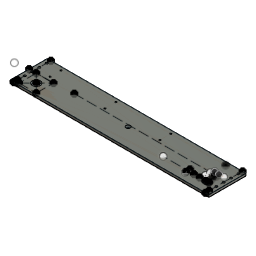
SideWall v52 (Autodesk Fusion 360 archive; units mm, degrees)
design "SideWall" references "tormach 770mx"
Autodesk Fusion 360 part; units mm, degrees
sketch "Sketch1" plane through (0, 0, 0) normal (0, 1, 0) x (1, 0, 0)
  line L0 (0, 0) -> (543, 0)
  line L1 (543, 0) -> (543, -101.6)
  line L2 (543, -101.6) -> (0, -101.6)
  line L3 (0, -101.6) -> (0, 0)
  dimension "d1" = 543
  dimension "d2" = 101.6
  constraint horizontal L0
  constraint vertical L1
  constraint horizontal L2
  constraint vertical L3
  constraint coincident L0.start L3.end
  measures "d1" distance of L0.start L0.end
  measures "d2" distance of L0.start L2.end
extrude "Extrude1" add sketch "Sketch1" along normal mid plane 6.35
sketch "Sketch2" plane through (0, 3.175, 0) normal (0, 1, 0) x (-1, 0, 0)
  line L0 (0, 101.6) -> (-543, 101.6)
  line L1 (-543, 101.6) -> (-543, 0)
  line L2 (-543, 0) -> (0, 0)
  line L3 (0, 0) -> (0, 101.6)
  line L4 (-534, 0) -> (-534, 101.6) construction
  line L5 (-10, 0) -> (-10, 101.6) construction
  line L6 (-506.5, 80.1) -> (-514.5, 80.1)
  arc A0 (-514.5, 80.1) -> (-514.5, 66.1) centre (-514.5, 73.1) ccw
  line L7 (-514.5, 66.1) -> (-506.5, 66.1)
  arc A1 (-506.5, 66.1) -> (-506.5, 80.1) centre (-506.5, 73.1) ccw
  line L8 (-506.5, 73.1) -> (-514.5, 73.1) construction
  line L9 (-506.5, 73.1) -> (-390, 73.1) construction
  line L10 (0, 49.6) -> (-66.57, 49.6) construction
  line L11 (-19.43, 96.67) -> (-66.57, 96.67) construction
  line L12 (-66.57, 96.67) -> (-66.57, 49.53) construction
  line L13 (-66.57, 49.53) -> (-19.43, 49.53) construction
  line L14 (-19.43, 49.53) -> (-19.43, 96.67) construction
  line L15 (-19.43, 96.67) -> (-66.57, 49.53) construction
  line L16 (-66.57, 96.67) -> (-19.43, 49.53) construction
  line L17 (-458, 67) -> (-458, 81) construction
  line L18 (-120, 46.09) -> (-504, 46.09) construction
  line L19 (-510, 47.46) -> (-510, 60.6) construction
  line L20 (-496.73, 39.09) -> (-522, 39.09) construction
  point P0 (-534, 91.6)
  point P1 (35, 55)
  point P2 (-10, 91.6)
  point P3 (-496.73, 9.09)
  point P4 (-496.73, 39.09)
  point P5 (-514.5, 73.1)
  point P6 (-506.5, 73.1)
  point P7 (-490, 73.1)
  point P8 (-474, 73.1)
  point P9 (-120, 46.09)
  point P10 (-504, 46.09)
  point P11 (-43, 73.1)
  point P12 (-19.43, 49.53)
  point P13 (-66.57, 49.53)
  point P14 (-66.57, 96.67)
  point P15 (-19.43, 96.67)
  point P16 (-458, 68.1)
  point P17 (-458, 78.1)
  point P18 (-508.73, 39.09)
  point P19 (-493, 60.6)
  point P20 (-493, 47.46)
  dimension "d6" = 10
  dimension "d14" = 10
  dimension "d15" = 10
  dimension "d27" = 30
  dimension "d40" = 8
  dimension "d42" = 28.5
  dimension "d43" = 14
  dimension "d45" = 16
  dimension "d46" = 490
  dimension "d47" = 506.5
  dimension "d48" = 534
  dimension "d49" = 496.73
  dimension "d50" = 92.51
  dimension "d68" = 52
  dimension "d69" = 120
  dimension "d70" = 504
  dimension "d77" = 47.14
  dimension "d78" = 47.14
  dimension "d79" = 43
  dimension "d80" = 28.5
  dimension "d102" = 10
  dimension "d103" = 16
  dimension "d104" = 5
  dimension "d112" = 55.51
  dimension "d114" = 510
  dimension "d115" = 13.14
  dimension "d122" = 41
  dimension "d123" = 12
  constraint coincident L2 L4.start
  constraint coincident L0 L4.end
  constraint perpendicular L0 L4
  constraint coincident L4 P0
  constraint coincident L2 L5.start
  constraint coincident L0 L5.end
  constraint perpendicular L0 L5
  constraint coincident L5 P2
  constraint horizontal P5 P6
  constraint tangent L6 A0
  constraint tangent A0 L7
  constraint parallel L6 L7
  constraint tangent L7 A1
  constraint tangent L6 A1
  constraint coincident P5 A0.centre
  constraint horizontal L8
  constraint coincident P6 A1.centre
  constraint parallel L8 L9
  constraint coincident L9 P7
  constraint coincident L9 P8
  constraint coincident L3 L10.start
  constraint horizontal L11
  constraint perpendicular L11 L12
  constraint parallel L11 L13
  constraint parallel L12 L14
  constraint coincident L15 P11
  constraint coincident L16 P11
  constraint coincident P12 L13.end
  constraint coincident P13 L12.end
  constraint coincident P14 L11.end
  constraint coincident P15 L11.start
  constraint perpendicular L9 L17
  constraint coincident L17 P16
  constraint coincident L17 P17
  constraint coincident L12 L10.end
  constraint coincident P9 L18.start
  constraint coincident P10 L18.end
  constraint parallel L9 L18
  constraint vertical L19.start L19.end
  constraint coincident P4 L20.start
  constraint perpendicular L1 L20
  constraint coincident L20 P18
  measures "d6" distance of L0 P0
  measures "d14" distance of L3 L5
  measures "d15" distance of L0 P2
  measures "d27" distance of P3 P4
  measures "d40" distance of P5 P6
  measures "d42" distance of L0 P5
  measures "d43" diameter of A0
  measures "d45" distance of P7 P8
  measures "d46" distance of L3 P7
  measures "d47" distance of L3 P6
  measures "d48" distance of L3 P0
  measures "d49" distance of L3 P3
  measures "d50" distance of L0 P3
  measures "d68" distance of L0 L10
  measures "d69" distance of L3 P9
  measures "d70" distance of L3 P10
  measures "d77" distance of P13 P12
  measures "d78" distance of P14 P13
  measures "d79" distance of L3 P11
  measures "d80" distance of L0 P11
  measures "d102" distance of P16 P17
  measures "d103" distance of P8 L17
  measures "d104" distance of L9 P17
  measures "d112" distance of L0 L18
  measures "d114" distance of L3 L19.end
  measures "d115" distance of L19.start L19.end
  measures "d122" distance of L0 L19.end
  measures "d123" distance of P4 P18
hole "Hole1" at (534, 3.175, 91.6) direction (0, -1, 0) diameter 6 end through all
pattern_linear "R-Pattern1" count 1 spacing 0 along (-1, 0, 0) count 5 spacing 20 along (0, 0, -1) of "Hole1"
hole "Hole5" at (496.73, 3.175, 9.09) direction (0, -1, 0) diameter 4.2 end through all
hole "Hole6" at (496.73, 3.175, 39.09) direction (0, -1, 0) diameter 4.3 end through all
pattern_linear "R-Pattern2" count 1 spacing 0 along (0, 0, 1) count 4 spacing 150 along (-1, 0, 0) of "Hole5", "Hole6"
extrude "Extrude2" cut sketch "Sketch2" along normal through all and the other way through all contours L6 A0 L7 A1
hole "Hole7" at (10, 3.175, 91.6) direction (0, -1, 0) diameter 6 end through all
pattern_linear "R-Pattern4" count 1 spacing 0 along (1, 0, 0) count 5 spacing 20 along (0, 0, -1) of "Hole7"
hole "Hole8" at (490, 3.175, 73.1) direction (0, -1, 0) diameter 3.3 end through all
hole "Hole9" at (474, 3.175, 73.1) direction (0, -1, 0) diameter 3.3 end through all
hole "Hole10" at (120, 3.175, 46.09) direction (0, -1, 0) diameter 3.4 end through all
hole "Hole11" at (504, 3.175, 46.09) direction (0, -1, 0) diameter 3.4 end through all
hole "Hole12" at (43, 3.175, 73.1) direction (0, -1, 0) diameter 22.1 end through all
hole "Hole13" at (19.43, 3.175, 49.53) direction (0, -1, 0) diameter 3.3 end through all
hole "Hole14" at (66.57, 3.175, 49.53) direction (0, -1, 0) diameter 3.3 depth 12.7 tip angle 118
hole "Hole15" at (66.57, 3.175, 96.67) direction (0, -1, 0) diameter 3.3 depth 12.7 tip angle 118
hole "Hole16" at (19.43, 3.175, 96.67) direction (0, -1, 0) diameter 3.3 depth 12.7 tip angle 118
hole "Hole17" at (458, 3.175, 68.1) direction (0, -1, 0) diameter 2.5 end through all
hole "Hole18" at (458, 3.175, 78.1) direction (0, -1, 0) diameter 2.5 depth 12.7 tip angle 118
hole "Hole19" at (510, 3.175, 47.46) direction (0, -1, 0) diameter 2.5 end through all
hole "Hole20" at (510, 3.175, 60.6) direction (0, -1, 0) diameter 2.8 end through all
hole "Hole21" at (508.73, 3.175, 39.09) direction (0, -1, 0) diameter 2.5 end through all
sketch "Sketch3" plane through (0, 3.175, 0) normal (0, 1, 0) x (-1, 0, 0)
  line L0 (-562, 50.75) -> (18, 50.75) construction
  line L1 (-272, 100) -> (-272, 0) construction
  line L2 (0, 0) -> (0, 101.6)
  line L3 (-543, 0) -> (0, 0)
  point P0 (-272, 50.75)
  dimension "d133" = 272
  dimension "d134" = 50.75
  constraint horizontal L0
  constraint perpendicular L0 L1
  constraint midpoint L0 P0
  measures "d133" distance of L1 L2
  measures "d134" distance of L0 L3
hole "Hole23" at (272, 3.175, 50.75) direction (0, -1, 0) diameter 12 end through all
hole "Hole24" at (493, 3.175, 60.6) direction (0, -1, 0) diameter 2.8 end through all
hole "Hole25" at (493, 3.175, 47.46) direction (0, -1, 0) diameter 2.5 depth 6.35 tip angle 118
